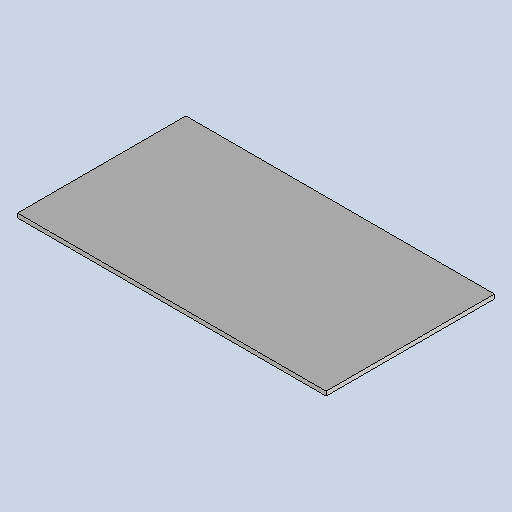
# Autodesk Inventor part: PNS-633 charging blind flange
Saved by Autodesk Inventor 2025.1 (Build 291241020, 241B)
## iProperties
Created: 2025-02-13
Part Number: PNS-633 charging blind flange
Material: Generic
Document SubType Name: Sheet Metal
Designer: pokla
Density: 1 g/cm^3
Sheet Metal Rule: Default
Sheet Metal Width: 0,000 mm
Sheet Metal Length: 0,000 mm
Sheet Metal Area: 0,000 mm^2
Appearance: Default
Author: pokla
Autodesk Inventor part; units mm, degrees
ref_plane "YZ Plane" through (0, 0, 0) normal (1, 0, 0) x (0, 1, 0)
ref_plane "XZ Plane" through (0, 0, 0) normal (0, 1, 0) x (-1, 0, 0)
ref_plane "XY Plane" through (0, 0, 0) normal (0, 0, 1) x (1, 0, 0)
sketch "Sketch4" plane through (0, 0, 0) normal (0, 0, 1) x (1, 0, 0)
  line L0 (-110, 60) -> (110, 60)
  line L1 (110, 60) -> (110, -60)
  line L2 (110, -60) -> (-110, -60)
  line L3 (-110, -60) -> (-110, 60)
  line L4 (-110, 60) -> (110, -60) construction
  line L5 (110, 60) -> (-110, -60) construction
  point P0 (0, 0)
  dimension "Charging_hatch_lenght" = 120
  dimension "d12" = 120
  dimension "d13" = 220
  measures "d12" distance of L0.end L1.end
  measures "d13" distance of L1.end L2.end
extrude "Plate2" add sketch "Sketch4" along normal blind 3.048
equation "\"d12\" = Charging_hatch_lenght"
equation "\"d13\" = Charging_hatch_width - Charging_hatch_hight"
equation "\"d14\" = Thickness"
equation "\"BendRadius\" = Thickness"
equation "\"BendReliefWidth\" = Thickness"
equation "\"BendReliefDepth\" = 0.5 * Thickness"
equation "\"CornerReliefSize\" = 4 * Thickness"
equation "\"MinimumRemnant\" = 2 * Thickness"
equation "\"TransitionRadius\" = BendRadius"
equation "\"JacobiRadiusSize\" = BendRadius"
equation "\"GapSize\" = Thickness"
equation "\"Charging_hatch_width\" = 400"
equation "\"Charging_hatch_hight\" = 180"
equation "\"Thickness\" = 3.048"
body "Solid3"
